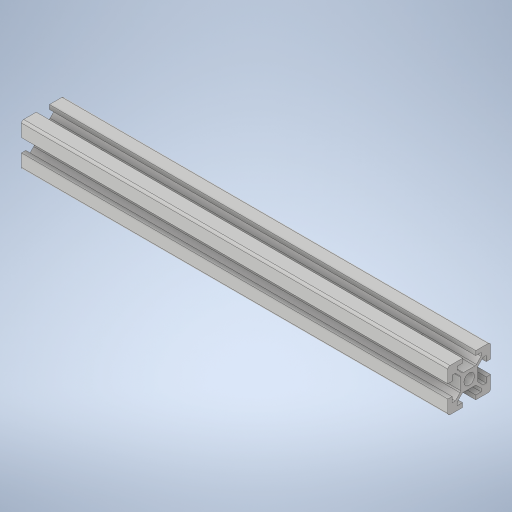
# Autodesk Inventor part: Perfil 200
Saved by Autodesk Inventor 2024.2 (Build 282272000, 272)
## iProperties
Created: 2023-10-26
Part Number: Perfil 200
Material: Generic
Document SubType Name: Modeling
Designer: lugomez
Density: 1 g/cm^3
Appearance: Default
Author: lugomez
Autodesk Inventor part; units mm, degrees
ref_plane "YZ Plane" through (0, 0, 0) normal (1, 0, 0) x (0, 1, 0)
ref_plane "XZ Plane" through (0, 0, 0) normal (0, 1, 0) x (-1, 0, 0)
ref_plane "XY Plane" through (0, 0, 0) normal (0, 0, 1) x (1, 0, 0)
sketch "Sketch1" plane through (0, 0, 0) normal (1, 0, 0) x (0, 1, 0)
  circle A0 centre (0, 0) radius 2.5
  line L0 (-10, -10) -> (10, 10) construction
  line L1 (10, -10) -> (-10, 10) construction
  line L2 (10, 3.1) -> (8, 3.1)
  line L3 (8, 3.1) -> (8, 5.6)
  line L4 (8, 5.6) -> (6.5, 5.6)
  line L5 (6.5, 5.6) -> (4, 3.1)
  line L6 (4, 3.1) -> (4, -3.1)
  line L7 (4, -3.1) -> (6.5, -5.6)
  line L8 (6.5, -5.6) -> (8, -5.6)
  line L9 (8, -5.6) -> (8, -3.1)
  line L10 (8, -3.1) -> (10, -3.1)
  line L11 (10, -9) -> (10, -3.1)
  line L12 (10, 3.1) -> (10, 9)
  line L13 (-3.1, 10) -> (-3.1, 8)
  line L14 (-3.1, 8) -> (-5.6, 8)
  line L15 (-5.6, 8) -> (-5.6, 6.5)
  line L16 (-5.6, 6.5) -> (-3.1, 4)
  line L17 (-3.1, 4) -> (3.1, 4)
  line L18 (3.1, 4) -> (5.6, 6.5)
  line L19 (5.6, 6.5) -> (5.6, 8)
  line L20 (5.6, 8) -> (3.1, 8)
  line L21 (3.1, 8) -> (3.1, 10)
  line L22 (-10, -3.1) -> (-8, -3.1)
  line L23 (-8, -3.1) -> (-8, -5.6)
  line L24 (-8, -5.6) -> (-6.5, -5.6)
  line L25 (-6.5, -5.6) -> (-4, -3.1)
  line L26 (-4, -3.1) -> (-4, 3.1)
  line L27 (-4, 3.1) -> (-6.5, 5.6)
  line L28 (-6.5, 5.6) -> (-8, 5.6)
  line L29 (-8, 5.6) -> (-8, 3.1)
  line L30 (-8, 3.1) -> (-10, 3.1)
  line L31 (3.1, -10) -> (3.1, -8)
  line L32 (3.1, -8) -> (5.6, -8)
  line L33 (5.6, -8) -> (5.6, -6.5)
  line L34 (5.6, -6.5) -> (3.1, -4)
  line L35 (3.1, -4) -> (-3.1, -4)
  line L36 (-3.1, -4) -> (-5.6, -6.5)
  line L37 (-5.6, -6.5) -> (-5.6, -8)
  line L38 (-5.6, -8) -> (-3.1, -8)
  line L39 (-3.1, -8) -> (-3.1, -10)
  line L40 (-9, -10) -> (-3.1, -10)
  line L41 (3.1, -10) -> (9, -10)
  line L42 (-10, 9) -> (-10, 3.1)
  line L43 (-10, -3.1) -> (-10, -9)
  line L44 (9, 10) -> (3.1, 10)
  line L45 (-3.1, 10) -> (-9, 10)
  arc A1 (10, 9) -> (9, 10) centre (9, 9) ccw
  arc A2 (-9, 10) -> (-10, 9) centre (-9, 9) ccw
  arc A3 (-10, -9) -> (-9, -10) centre (-9, -9) ccw
  arc A4 (9, -10) -> (10, -9) centre (9, -9) ccw
  dimension "d1" = 20
  dimension "d3" = 6.2
  dimension "d4" = 3.1
  dimension "d6" = 11.2
  dimension "d7" = 5.6
  dimension "d8" = 4
  dimension "d9" = 5
  dimension "d10" = 45
  dimension "d11" = 45
  dimension "d12" = 1.5
  dimension "d15" = 360
  dimension "d17" = 10
  dimension "d18" = 2
  dimension "d21" = 1
  constraints: 92 end point, 16 point on line, 10 parallel, 10 perpendicular, 8 point on circle, 8 tangent, 5 centre point, 3 equal radius, 2 horizontal, 2 midpoint, 1 coincident, 1 vertical alignment, 77 other
  measures "d1" distance of L1.start L0.end
  measures "d3" distance between parallel lines of L10 L2
  measures "d4" distance from line of L2 point (0, 0)
  measures "d6" distance between parallel lines of L4 L8
  measures "d7" distance from line of L4 point (0, 0)
  measures "d8" distance from line of L6 point (0, 0)
  measures "d9" diameter of A0
  measures "d10" angle of L5 L6
  measures "d11" angle of L6 L7
  measures "d12" distance of L3.end L4.end
  measures "d17" distance from line of A0.centre L11
  measures "d18" distance between parallel lines of L11 L9
  measures "d21" radius of A1
extrude "300" add sketch "Sketch1" against normal blind 200
fillet "Fillet1" radius 1 8 edges at (-100, 4, 3.1) (-100, 4, -3.1) (-100, -4, 3.1) (-100, -4, -3.1) (-100, 3.1, 4) (-100, -3.1, 4) (-100, -3.1, -4) (-100, 3.1, -4)
sketch "Boceto2" plane through (0, 4, 2.6858) normal (0, 1, 0) x (1, 0, 0)
  circle A0 centre (-175, 2.6858) radius 3
  circle A1 centre (-25, 2.6858) radius 3
  line L0 (0, 5.3716) -> (0, 0) projected
  line L1 (-200, 0) -> (-200, 5.3716) projected
  point P0 (0, 2.6858)
  point P1 (0, 2.6858)
  point P2 (-200, 2.6858)
  dimension "d23" = 25
  dimension "d24" = 6
  dimension "d25" = 25
  constraints: 2 centre point, 2 horizontal alignment, 2 midpoint, 1 equal radius
  measures "d23" distance from line of L1 A0.centre
  measures "d24" diameter of A0
  measures "d25" distance from line of L0 A1.centre
extrude "Extrusión2" cut sketch "Boceto2" against normal through all
equation "\"d4\" = 0.5 * d3"
equation "\"d7\" = 0.5 * d6"
equation "\"d11\" = d10"
equation "\"d25\" = d23"
body "Solid1"
